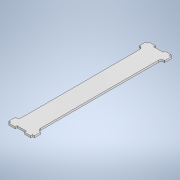
# Autodesk Inventor part: camRiser
Saved by Autodesk Inventor 2020 (Build 240168000, 168)
## iProperties
Created: 2019-08-06
Part Number: camRiser
Material: Generic
Document SubType Name: Modeling
Designer: n10208577
Density: 1 g/cm^3
Appearance: Default
Author: n10208577
Autodesk Inventor part; units mm, degrees
ref_plane "YZ Plane" through (0, 0, 0) normal (1, 0, 0) x (0, 1, 0)
ref_plane "XZ Plane" through (0, 0, 0) normal (0, 1, 0) x (-1, 0, 0)
ref_plane "XY Plane" through (0, 0, 0) normal (0, 0, 1) x (1, 0, 0)
sketch "Sketch1" plane through (0, 0, 0) normal (0, 1, 0) x (-1, 0, 0)
  line L0 (-5.0543, -97.83) -> (-5.0543, 92.17)
  arc A0 (-10.0543, -102.83) -> (-5.0543, -97.83) centre (-10.0543, -97.83) ccw
  arc A1 (-5.0543, 92.17) -> (-10.0543, 97.17) centre (-10.0543, 92.17) ccw
  line L1 (24.9457, 92.17) -> (24.9457, -97.83)
  line L2 (17.4457, -112.83) -> (17.4457, -115.83)
  line L3 (17.4457, -115.83) -> (27.4457, -115.83)
  line L4 (27.4457, -115.83) -> (27.4457, -112.83)
  line L5 (2.4457, -112.83) -> (2.4457, -115.83)
  line L6 (2.4457, -115.83) -> (-7.5543, -115.83)
  line L7 (-7.5543, -115.83) -> (-7.5543, -112.83)
  line L8 (2.4457, -112.83) -> (17.4457, -112.83)
  line L9 (-7.5543, -112.83) -> (-10.5543, -112.83)
  line L10 (-10.5543, -112.83) -> (-10.5543, -102.83)
  line L11 (-10.5543, -102.83) -> (-10.0543, -102.83)
  line L12 (27.4457, -112.83) -> (30.4457, -112.83)
  line L13 (30.4457, -112.83) -> (30.4457, -102.83)
  line L14 (30.4457, -102.83) -> (29.9457, -102.83)
  arc A2 (24.9457, -97.83) -> (29.9457, -102.83) centre (29.9457, -97.83) ccw
  line L15 (2.4457, 107.17) -> (2.4457, 110.17)
  line L16 (2.4457, 110.17) -> (-7.5543, 110.17)
  line L17 (-7.5543, 110.17) -> (-7.5543, 107.17)
  line L18 (17.4457, 107.17) -> (17.4457, 110.17)
  line L19 (17.4457, 110.17) -> (27.4457, 110.17)
  line L20 (27.4457, 110.17) -> (27.4457, 107.17)
  line L21 (17.4457, 107.17) -> (2.4457, 107.17)
  line L22 (27.4457, 107.17) -> (30.4457, 107.17)
  line L23 (30.4457, 107.17) -> (30.4457, 97.17)
  line L24 (30.4457, 97.17) -> (29.9457, 97.17)
  arc A3 (29.9457, 97.17) -> (24.9457, 92.17) centre (29.9457, 92.17) ccw
  line L25 (-7.5543, 107.17) -> (-10.5543, 107.17)
  line L26 (-10.5543, 107.17) -> (-10.5543, 97.17)
  line L27 (-10.5543, 97.17) -> (-10.0543, 97.17)
  point P0 (0, 0)
  constraints: 56 end point, 8 point on circle, 4 centre point
extrude "Extrusion1" add sketch "Sketch1" along normal blind 3
body "Solid1"
